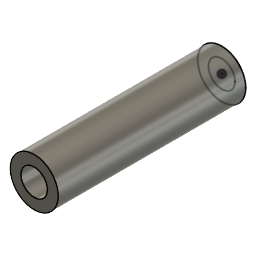
bujes_rigidez (Autodesk Fusion 360 design; units mm, degrees)
part number: 2026-03-20-21-01-39-227
Autodesk Fusion 360 part; units mm, degrees
sketch "Boceto1" plane through (0, 0, 0) normal (0, 0, 1) x (1, 0, 0)
  circle A0 centre (0, 0) radius 5
  circle A1 centre (0, 0) radius 2.75
  dimension "d1" = 10
  dimension "d2" = 5.5
  constraint coincident A0.centre A1.centre
  constraint concentric A0 A1
  measures "d1" diameter of A0
  measures "d2" diameter of A1
extrude "Extruir1" add sketch "Boceto1" along normal blind 39
